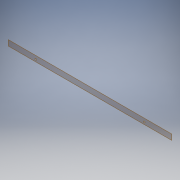
# Autodesk Inventor part: Lateral 1 Gaveta
Saved by Autodesk Inventor 2018 (Build 220112000, 112)
## iProperties
Created: 2018-07-09
Part Number: Lateral 1 Gaveta
Material: PMMA plástico
Document SubType Name: Chapa de metal
Designer: Regner
Density: 1.188 g/cm^3
Sheet Metal Rule: Padrão_mm
Appearance: Policarbonato - Fumê
Author: Regner
Autodesk Inventor part; units mm, degrees
ref_plane "YZ Plane" through (0, 0, 0) normal (1, 0, 0) x (0, 1, 0)
ref_plane "XZ Plane" through (0, 0, 0) normal (0, 1, 0) x (-1, 0, 0)
ref_plane "XY Plane" through (0, 0, 0) normal (0, 0, 1) x (1, 0, 0)
sketch "Esboço1" plane through (0, 0, 0) normal (0, 1, 0) x (-1, 0, 0)
  line L0 (149, 5) -> (-149, 5)
  line L1 (-149, 5) -> (-149, -5)
  line L2 (-149, -5) -> (149, -5)
  line L3 (149, -5) -> (149, 5)
  line L4 (149, 5) -> (-149, -5) construction
  line L5 (-149, 5) -> (149, -5) construction
  point P0 (0, 0)
  dimension "d0" = 298
  dimension "d1" = 10
  measures "d0" distance of L2.end L1.end
  measures "d1" distance of L0.end L1.end
extrude "Placa1" add sketch "Esboço1" along normal blind 0.5
sketch "Esboço2" plane through (0, 0, 0) normal (0, -1, 0) x (1, 0, 0)
  line L0 (149, -5) -> (-149, -5) projected
  line L1 (149, 5) -> (149, -5) projected
  line L2 (-149, -5) -> (-149, 5) projected
  point P0 (0, 0)
  point P1 (-99, -1)
  point P2 (99, -1)
  dimension "d3" = 4
  dimension "d4" = 4
  dimension "d5" = 50
  dimension "d6" = 50
  measures "d3" distance from line of L0 point (-99, -1)
  measures "d4" distance from line of L0 point (99, -1)
  measures "d5" distance from line of L1 point (99, -1)
  measures "d6" distance from line of L2 point (-99, -1)
hole "Furo1" at (-99, 0, -1) at (99, 0, -1) direction (0, 1, 0) diameter 3 end through all
equation "\"d12\" = Espessura"
equation "\"d2\" = Espessura"
equation "\"Raio_vergadura\" = Espessura"
equation "\"Largura_alívio_de_vergadura\" = Espessura"
equation "\"Profundidade_alívio_de_vergadura\" = 0.5 * Espessura"
equation "\"Tamanho_alívio_de_dobra\" = 4 * Espessura"
equation "\"Remanescente_mínimo\" = 2 * Espessura"
equation "\"Raiodetransição\" = Raio_vergadura"
equation "\"Tamanho_de_raio_de_Jacobi\" = Raio_vergadura"
equation "\"TamanhoFolga\" = Espessura"
equation "\"Espessura\" = 0.5"
